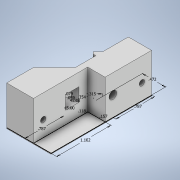
# Autodesk Inventor part: minimal micro scanner
Saved by Autodesk Inventor 2022 (Build 260153000, 153)
## iProperties
Created: 2023-06-22
Part Number: minimal micro scanner
Material: Generic
Document SubType Name: Modeling
Designer: William
Density: 1 g/cm^3
Appearance: Default
Author: William
Autodesk Inventor part; units mm, degrees
ref_plane "YZ Plane" through (0, 0, 0) normal (1, 0, 0) x (0, 1, 0)
ref_plane "XZ Plane" through (0, 0, 0) normal (0, 1, 0) x (-1, 0, 0)
ref_plane "XY Plane" through (0, 0, 0) normal (0, 0, 1) x (1, 0, 0)
sketch "Sketch1" plane through (0, 0, 0) normal (0, 1, 0) x (-1, 0, 0)
  line L0 (0, 0) -> (22.8388, 0)
  line L1 (22.8388, 0) -> (22.8388, -52)
  line L2 (22.8388, -52) -> (0, -52)
  line L3 (0, -52) -> (0, 0)
  line L4 (9, 0) -> (9, -16.4645)
  line L5 (12, -24.5962) -> (12, -35.182)
  line L6 (9, -28) -> (0, -28)
  line L7 (12, -35.182) -> (13.4142, -35.182)
  line L8 (13.4142, -35.182) -> (19.7782, -28.818)
  line L9 (19.7782, -28.818) -> (20.8388, -29.8787)
  line L10 (20.8388, -29.8787) -> (12, -38.7175)
  line L11 (12, -38.7175) -> (12, -52)
  line L12 (16.5962, -32) -> (17.6569, -33.0607) construction
  line L13 (16.5962, -32) -> (0, -32) construction
  line L14 (9, -16.4645) -> (9, -28)
  line L15 (20.8388, -29.8787) -> (19.7782, -28.818)
  line L16 (12, -24.5962) -> (21.1924, -15.4038)
  line L17 (16.5962, -32) -> (16.5962, -20) construction
  line L18 (16.5962, -20) -> (9, -20) construction
  line L19 (21.1924, -15.4038) -> (22.8388, -13.7574)
  line L20 (20.8388, -29.8787) -> (22.8388, -27.8787)
  line L21 (19.7782, -28.818) -> (22.8388, -25.7574)
  dimension "d8" = 9
  dimension "d9" = 1.5
  dimension "d10" = 8
  dimension "d11" = 20
  dimension "d12" = 12
  dimension "d18" = 28
  dimension "d46" = 45
  dimension "d48" = 3
  dimension "d49" = 45
  dimension "d50" = 2
  dimension "d51" = 4
  dimension "d52" = 20
  constraints: 44 end point, 9 point on line, 6 perpendicular, 4 collinear, 3 parallel, 3 vertical, 2 horizontal, 2 midpoint, 1 vertical alignment
  measures "d8" distance of L7.end L8.end
  measures "d9" distance of L8.end L9.end
  measures "d10" distance of L10.end L12.end
  measures "d11" distance between parallel lines of L2 L13
  measures "d12" distance between parallel lines of L3 L5
  measures "d18" distance between parallel lines of L6 L0
  measures "d46" angle of L17 L16
  measures "d48" distance between parallel lines of L5 L14
  measures "d49" angle of L17 L8
  measures "d50" distance from line of L1 L9.end
  measures "d51" distance between parallel lines of L6 L13
  measures "d52" distance between parallel lines of L0 L18
extrude "Extrusion2" add sketch "Sketch1" along normal blind 20 contours L0 L1 L19 L16 L5 L7 L8 L9 L10 L11 L2 L3 L6 L14 L4 | L1 L20 L9 L21
sketch "Sketch3" plane through (-9, 0, 0) normal (1, 0, 0) x (0, 0, -1)
  line L0 (0, 0) -> (0, 20) projected
  line L1 (23.5, 13.5) -> (16.5, 13.5)
  line L2 (16.5, 13.5) -> (16.5, 6.5)
  line L3 (16.5, 6.5) -> (23.5, 6.5)
  line L4 (23.5, 6.5) -> (23.5, 13.5)
  circle A0 centre (5, 8) radius 1.397
  point P0 (16.5, 10)
  point P1 (16.5, 10)
  point P2 (0, 10)
  point P3 (20, 0)
  point P4 (20, 0)
  point P5 (20, 0)
  point P6 (20, 6.5)
  point P7 (0, 10)
  dimension "d19" = 2.794
  dimension "d20" = 5
  dimension "d33" = 2
  dimension "d53" = 7
  constraints: 8 end point, 4 midpoint, 2 parallel, 2 perpendicular, 1 centre point, 1 coincident, 1 horizontal, 1 horizontal alignment, 1 vertical alignment
  measures "d19" diameter of A0
  measures "d20" distance from line of L0 A0.centre
  measures "d33" vertical distance of point (0, 10) A0.centre
  measures "d53" distance of L1.start L1.end
extrude "Extrusion3" cut sketch "Sketch3" against normal up to next
sketch "Sketch4" plane through (0, 0, -28) normal (1, 0, 0) x (0, 0, -1)
  line L0 (24, 0) -> (24, 20) projected
  circle A0 centre (19, 8) radius 1.397
  circle A1 centre (4, 10) radius 2
  circle A2 centre (4, 10) radius 1.05
  point P0 (-28, 0)
  point P1 (24, 10)
  point P2 (24, 10)
  dimension "d23" = 2.794
  dimension "d24" = 4
  dimension "d25" = 2.1
  dimension "d26" = 5
  dimension "d27" = 2
  dimension "d28" = 20
  constraints: 3 centre point, 2 midpoint, 1 coincident, 1 horizontal alignment
  measures "d23" diameter of A0
  measures "d24" diameter of A1
  measures "d25" diameter of A2
  measures "d26" horizontal distance of A0.centre point (24, 10)
  measures "d27" vertical distance of point (24, 10) A0.centre
  measures "d28" distance of point (24, 10) A1.centre
extrude "Extrusion4" cut sketch "Sketch4" against normal up to next contours A0 | A2
extrude "Extrusion5" cut sketch "Sketch4" against normal blind 9 contours A1
sketch "Sketch5" plane through (-20.8388, 0, -29.8787) normal (-0.7071068, 0, -0.7071068) x (-0.7071068, 0, 0.7071068)
  ellipse E0 centre (-7.75, 10) end of major axis (-7.75, 11.05) minor radius 0.7425 projected
  line L0 (-10.5, 4) -> (1.5, 4) construction
  line L1 (1.5, 4) -> (1.5, 16) construction
  line L2 (1.5, 16) -> (-10.5, 16) construction
  line L3 (-10.5, 16) -> (-10.5, 4) construction
  circle A0 centre (-10.5, 16) radius 0.5
  circle A1 centre (-10.5, 4) radius 0.5
  line L4 (-9, 5.5) -> (5.0245, 5.5)
  line L5 (5.0245, 5.5) -> (5.0245, 21.8088)
  line L6 (5.0245, 21.8088) -> (-9, 21.8088)
  line L7 (-9, 21.8088) -> (-9, 5.5)
  circle A2 centre (1.5, 4) radius 0.5
  point P0 (6.3921, 0)
  point P1 (-4.5, 0)
  point P2 (-4.5, 0)
  point P3 (-4.5, 0)
  point P4 (-10.5, 10)
  point P5 (-4.5, 4)
  point P6 (-4.5, 10)
  dimension "d35" = 12
  dimension "d37" = 1
  dimension "d40" = 4.5
  dimension "d41" = 4.5
  constraints: 16 end point, 4 parallel, 3 centre point, 3 coincident, 3 perpendicular, 2 equal radius, 2 horizontal, 2 horizontal alignment, 2 midpoint, 2 vertical alignment, 1 other
  measures "d35" distance of L0.end L1.end
  measures "d37" diameter of A1
  measures "d40" distance from line of L7 point (-4.5, 10)
  measures "d41" distance from line of L4 point (-4.5, 10)
extrude "Extrusion6" cut sketch "Sketch5" against normal blind 3.5 contours E0 | A0 | A1 | L7 L6 L5 L4 | A2
extrude "Extrusion1" add sketch "Sketch1" against normal blind 3
chamfer "Chamfer1" distance 2.54 angle 45 4 edges at (-22.8388, -3, -26) (-11.4194, -3, -52) (-11.4194, -3, 0) (0, -3, -26)
body "Solid1"
